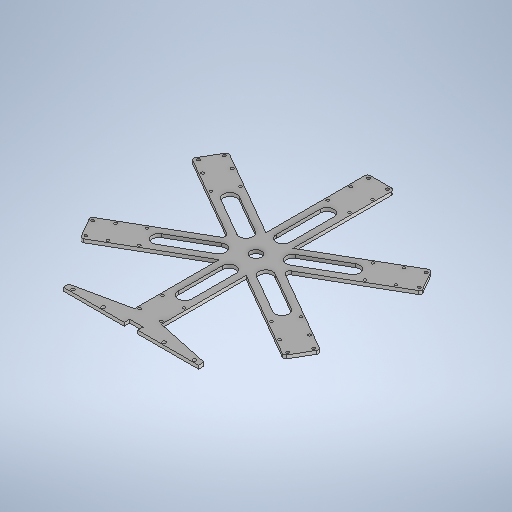
# Autodesk Inventor part: 03
Saved by Autodesk Inventor 2025.1 (Build 291241000, 241)
## iProperties
Created: 2024-09-17
Part Number: 03
Material: Generisch
Document SubType Name: Modeling
Designer: ffogue
Density: 1 g/cm^3
Appearance: Vorgabe
Author: ffogue
Autodesk Inventor part; units mm, degrees
ref_plane "YZ Plane" through (0, 0, 0) normal (1, 0, 0) x (0, 1, 0)
ref_plane "XZ Plane" through (0, 0, 0) normal (0, 1, 0) x (-1, 0, 0)
ref_plane "XY Plane" through (0, 0, 0) normal (0, 0, 1) x (1, 0, 0)
sketch "Sketch1" plane through (0, 0, 0) normal (0, 0, 1) x (1, 0, 0)
  line L0 (-100, 0) -> (-100, -8)
  line L1 (-100, -8) -> (100, -8)
  line L2 (100, -8) -> (100, 0)
  line L3 (0, 0) -> (0, 177) construction
  line L4 (0, 177) -> (82.7625, 129.217) construction
  line L5 (0, 177) -> (-160.2147, 269.5) construction
  line L6 (0, 177) -> (160.2147, 269.5) construction
  line L7 (0, 177) -> (0, 205.8158) construction
  line L8 (0, 177) -> (-85.2909, 127.7573) construction
  line L9 (94.0747, 177) -> (-94.0747, 177) construction
  circle A0 centre (0, 177) radius 40 construction
  line L10 (0, 137) -> (0, 72) construction
  line L11 (10, 137) -> (10, 72)
  line L12 (-10, 72) -> (-10, 137)
  arc A1 (10, 137) -> (-10, 137) centre (0, 137) ccw
  arc A2 (-10, 72) -> (10, 72) centre (0, 72) ccw
  line L13 (-34.641, 157) -> (-90.9327, 124.5) construction
  line L14 (-39.641, 165.6603) -> (-95.9327, 133.1603)
  line L15 (-85.9327, 115.8397) -> (-29.641, 148.3397)
  arc A3 (-29.641, 148.3397) -> (-39.641, 165.6603) centre (-34.641, 157) ccw
  arc A4 (-95.9327, 133.1603) -> (-85.9327, 115.8397) centre (-90.9327, 124.5) ccw
  line L16 (-34.641, 197) -> (-90.9327, 229.5) construction
  line L17 (-39.641, 188.3397) -> (-95.9327, 220.8397)
  line L18 (-85.9327, 238.1603) -> (-29.641, 205.6603)
  arc A5 (-39.641, 188.3397) -> (-29.641, 205.6603) centre (-34.641, 197) ccw
  arc A6 (-85.9327, 238.1603) -> (-95.9327, 220.8397) centre (-90.9327, 229.5) ccw
  line L19 (0, 217) -> (0, 282) construction
  line L20 (10, 217) -> (10, 282)
  line L21 (-10, 282) -> (-10, 217)
  arc A7 (-10, 217) -> (10, 217) centre (0, 217) ccw
  arc A8 (10, 282) -> (-10, 282) centre (0, 282) ccw
  line L22 (34.641, 197) -> (90.9327, 229.5) construction
  line L23 (39.641, 188.3397) -> (95.9327, 220.8397)
  line L24 (85.9327, 238.1603) -> (29.641, 205.6603)
  arc A9 (29.641, 205.6603) -> (39.641, 188.3397) centre (34.641, 197) ccw
  arc A10 (95.9327, 220.8397) -> (85.9327, 238.1603) centre (90.9327, 229.5) ccw
  line L25 (34.641, 157) -> (90.9327, 124.5) construction
  line L26 (29.641, 148.3397) -> (85.9327, 115.8397)
  line L27 (95.9327, 133.1603) -> (39.641, 165.6603)
  arc A11 (39.641, 165.6603) -> (29.641, 148.3397) centre (34.641, 157) ccw
  arc A12 (85.9327, 115.8397) -> (95.9327, 133.1603) centre (90.9327, 124.5) ccw
  circle A13 centre (0, 177) radius 105 construction
  line L28 (-20, 17) -> (-20, 142.359)
  line L29 (-20, 17) -> (-100, 0)
  line L30 (20, 17) -> (20, 142.359)
  line L31 (20, 17) -> (100, 0)
  arc A14 (-20, 142.359) -> (-20, 142.359) centre (-17.5, 138.0289) ccw
  line L32 (-20, 142.359) -> (-150.2147, 67.1795)
  line L33 (-150.2147, 67.1795) -> (-170.2147, 101.8205)
  line L34 (-170.2147, 101.8205) -> (-47.5, 172.6699)
  arc A15 (-47.5, 172.6699) -> (-47.5, 181.3301) centre (-50, 177) ccw
  line L35 (-170.2147, 252.1795) -> (-150.2147, 286.8205)
  arc A16 (-20, 211.641) -> (-20, 211.641) centre (-25, 211.641) ccw
  line L36 (-20, 211.641) -> (-20, 362)
  line L37 (-20, 362) -> (20, 362)
  line L38 (20, 362) -> (20, 211.641)
  line L39 (20, 211.641) -> (150.2147, 286.8205)
  line L40 (150.2147, 286.8205) -> (170.2147, 252.1795)
  line L41 (170.2147, 252.1795) -> (47.5, 181.3301)
  arc A17 (47.5, 181.3301) -> (47.5, 172.6699) centre (50, 177) ccw
  line L42 (47.5, 172.6699) -> (170.2147, 101.8205)
  line L43 (-170.2147, 252.1795) -> (-47.5, 181.3301)
  line L44 (-20, 211.641) -> (-150.2147, 286.8205)
  arc A18 (20, 142.359) -> (20, 142.359) centre (25, 142.359) ccw
  line L45 (20, 142.359) -> (150.2147, 67.1795)
  line L46 (150.2147, 67.1795) -> (170.2147, 101.8205)
  line L47 (0, 177) -> (160.2147, 84.5) construction
  line L48 (-10, -8) -> (-10, 0)
  line L49 (-10, 0) -> (10, 0)
  line L50 (10, 0) -> (10, -8)
  point P0 (0, 104.5)
  point P1 (-62.7868, 140.75)
  point P2 (-62.7868, 213.25)
  point P3 (0, 249.5)
  point P4 (62.7868, 213.25)
  point P5 (62.7868, 140.75)
  point P6 (20, 211.641)
  point P7 (-160.2147, 84.5)
  point P8 (0, 0)
  dimension "d10" = 80
  dimension "d0" = 200
  dimension "d1" = 8
  dimension "d4" = 60
  dimension "d6" = 60
  dimension "d7" = 60
  dimension "d8" = 60
  dimension "d9" = 185
  dimension "d11" = 10
  dimension "d12" = 10
  dimension "d13" = 10
  dimension "d14" = 10
  dimension "d15" = 10
  dimension "d16" = 10
  dimension "d17" = 210
  dimension "d19" = 25
  dimension "d20" = 25
  dimension "d21" = 5
  dimension "d22" = 90
  dimension "d25" = 5
  dimension "d30" = 185
  dimension "d32" = 185
  dimension "d33" = 185
  dimension "d34" = 5
  dimension "d35" = 185
  dimension "d36" = 5
  dimension "d39" = 5
  dimension "d40" = 185
  dimension "d43" = 8
  dimension "d44" = 20
  dimension "d84" = 40
  dimension "d85" = 40
  dimension "d86" = 40
  dimension "d87" = 40
  dimension "d114" = 40
  constraints: 114 end point, 40 point on circle, 30 tangent, 18 centre point, 16 parallel, 14 point on line, 12 midpoint, 8 vertical, 6 perpendicular, 5 horizontal alignment, 3 coincident, 2 horizontal, 21 other
  measures "d0" distance of L0.end L1.end
  measures "d1" distance of L0.start L0.end
  measures "d4" angle of L4 L3
  measures "d6" angle of L6 L7
  measures "d7" angle of L3 L8
  measures "d8" angle of L7 L5
  measures "d9" distance from line of L3.end L1
  measures "d11" radius of A3
  measures "d12" radius of A1
  measures "d13" radius of A11
  measures "d14" radius of A9
  measures "d15" radius of A7
  measures "d16" radius of A5
  measures "d17" diameter of A13
  measures "d19" vertical distance of L30.start L1.end
  measures "d20" distance from line of L28.start L1
  measures "d21" radius of A14
  measures "d22" angle of L32 L33
  measures "d25" radius of A15
  measures "d30" distance from line of L9 L36.end
  measures "d32" distance of L5.end L3.end
  measures "d33" distance of point (-160.215, 84.5) A13.centre
  measures "d34" radius of A16
  measures "d35" distance of L3.end L6.end
  measures "d36" radius of A17
  measures "d39" radius of A18
  measures "d40" distance of L47.end L3.end
  measures "d43" distance between parallel lines of L1 L49
  measures "d44" distance of L48.end L49.end
  measures "d84" distance between parallel lines of L32 L34
  measures "d85" distance between parallel lines of L44 L43
  measures "d86" distance between parallel lines of L38 L36
  measures "d87" distance between parallel lines of L41 L39
  measures "d114" distance between parallel lines of L30 L28
extrude "Extrusion2" add sketch "Sketch1" along normal mid plane 5 contours L29 L28 A14 L32 L33 L34 A15 L43 L35 L44 A16 L36 L37 L38 L39 L40 L41 A17 L42 L46 L45 A18 L30 L31 L2 L1 L50 L49 L48 L0 | L28 A14 | A18 L45 | L44 A16 picked at (-17.1896, 138.26) picked at (23.5757, 142.474) picked at (-23.6127, 211.5125)
sketch "Sketch3" plane through (0, 0, 2.5) normal (0, 0, 1) x (1, 0, 0)
  line L0 (-100, -8) -> (-10, -8) projected
  line L1 (-10, -8) -> (-10, 0) projected
  line L2 (-10, 0) -> (10, 0) projected
  line L3 (10, 0) -> (10, -8) projected
  line L4 (10, -8) -> (100, -8) projected
  line L5 (100, -8) -> (100, 0) projected
  line L6 (100, 0) -> (20, 17) projected
  line L7 (20, 17) -> (20, 142.359) projected
  line L8 (20, 142.359) -> (150.2147, 67.1795) projected
  line L9 (150.2147, 67.1795) -> (170.2147, 101.8205) projected
  line L10 (170.2147, 101.8205) -> (47.5, 172.6699) projected
  arc A0 (47.5, 181.3301) -> (47.5, 172.6699) centre (50, 177) ccw projected
  line L11 (47.5, 181.3301) -> (170.2147, 252.1795) projected
  line L12 (170.2147, 252.1795) -> (150.2147, 286.8205) projected
  line L13 (150.2147, 286.8205) -> (20, 211.641) projected
  line L14 (20, 211.641) -> (20, 362) projected
  line L15 (20, 362) -> (-20, 362) projected
  line L16 (-20, 362) -> (-20, 211.641) projected
  line L17 (-20, 211.641) -> (-150.2147, 286.8205) projected
  line L18 (-150.2147, 286.8205) -> (-170.2147, 252.1795) projected
  line L19 (-170.2147, 252.1795) -> (-47.5, 181.3301) projected
  arc A1 (-47.5, 172.6699) -> (-47.5, 181.3301) centre (-50, 177) ccw projected
  line L20 (-47.5, 172.6699) -> (-170.2147, 101.8205) projected
  line L21 (-170.2147, 101.8205) -> (-150.2147, 67.1795) projected
  line L22 (-150.2147, 67.1795) -> (-20, 142.359) projected
  line L23 (-20, 142.359) -> (-20, 17) projected
  line L24 (-20, 17) -> (-100, 0) projected
  line L25 (-100, 0) -> (-100, -8) projected
  arc A2 (39.641, 165.6603) -> (29.641, 148.3397) centre (34.641, 157) ccw projected
  line L26 (39.641, 165.6603) -> (95.9327, 133.1603) projected
  arc A3 (85.9327, 115.8397) -> (95.9327, 133.1603) centre (90.9327, 124.5) ccw projected
  line L27 (85.9327, 115.8397) -> (29.641, 148.3397) projected
  arc A4 (29.641, 205.6603) -> (39.641, 188.3397) centre (34.641, 197) ccw projected
  line L28 (29.641, 205.6603) -> (85.9327, 238.1603) projected
  arc A5 (95.9327, 220.8397) -> (85.9327, 238.1603) centre (90.9327, 229.5) ccw projected
  line L29 (95.9327, 220.8397) -> (39.641, 188.3397) projected
  arc A6 (-10, 217) -> (10, 217) centre (0, 217) ccw projected
  line L30 (-10, 217) -> (-10, 282) projected
  arc A7 (10, 282) -> (-10, 282) centre (0, 282) ccw projected
  line L31 (10, 282) -> (10, 217) projected
  line L32 (-85.9327, 238.1603) -> (-29.641, 205.6603) projected
  arc A8 (-39.641, 188.3397) -> (-29.641, 205.6603) centre (-34.641, 197) ccw projected
  line L33 (-39.641, 188.3397) -> (-95.9327, 220.8397) projected
  arc A9 (-85.9327, 238.1603) -> (-95.9327, 220.8397) centre (-90.9327, 229.5) ccw projected
  arc A10 (-29.641, 148.3397) -> (-39.641, 165.6603) centre (-34.641, 157) ccw projected
  line L34 (-29.641, 148.3397) -> (-85.9327, 115.8397) projected
  arc A11 (-95.9327, 133.1603) -> (-85.9327, 115.8397) centre (-90.9327, 124.5) ccw projected
  line L35 (-95.9327, 133.1603) -> (-39.641, 165.6603) projected
  line L36 (-10, 72) -> (-10, 137) projected
  arc A12 (10, 137) -> (-10, 137) centre (0, 137) ccw projected
  line L37 (10, 137) -> (10, 72) projected
  arc A13 (-10, 72) -> (10, 72) centre (0, 72) ccw projected
  line L38 (-50, 177) -> (50, 177) construction
  line L39 (0, 217) -> (0, 137) construction
  circle A14 centre (0, 177) radius 123 construction
  circle A15 centre (0, 177) radius 157 construction
  circle A16 centre (0, 177) radius 181 construction
  point P0 (0, 0)
  point P1 (14, 20)
  point P2 (14, 54)
  point P3 (-14, 20)
  point P4 (-14, 54)
  point P5 (55, -8)
  point P6 (-14, 299.2007)
  point P7 (14, 299.2007)
  point P8 (-14, 333.3746)
  point P9 (14, 333.3746)
  point P10 (-14, 357.4578)
  point P11 (14, 357.4578)
  dimension "d47" = 246
  dimension "d48" = 314
  dimension "d49" = 362
  dimension "d50" = 28
  dimension "d51" = 34
  dimension "d52" = 14
  dimension "d53" = 28
  dimension "d54" = 14
  dimension "d55" = 28
  constraints: 6 coincident, 6 point on circle, 5 midpoint, 5 vertical alignment, 4 end point, 4 horizontal alignment, 3 centre point, 1 vertical
  measures "d47" diameter of A14
  measures "d48" diameter of A15
  measures "d49" diameter of A16
  measures "d50" vertical distance of point (55, -8) point (14, 20)
  measures "d51" distance of point (14, 54) point (14, 20)
  measures "d52" horizontal distance of A13.centre point (-14, 54)
  measures "d53" distance of point (14, 54) point (-14, 54)
  measures "d54" horizontal distance of A7.centre A16.start
  measures "d55" distance of A16.end A16.start
fillet "Fillet1" radius 4 10 edges at (20, 362, 0) (-20, 362, 0) (150.2147, 286.8205, 0) (170.2147, 252.1795, 0) (170.2147, 101.8205, 0) (150.2147, 67.1795, 0) (-150.2147, 67.1795, 0) (-170.2147, 101.8205, 0) (-170.2147, 252.1795, 0) (-150.2147, 286.8205, 0)
sketch "Sketch4" plane through (0, 0, 2.5) normal (0, 0, 1) x (1, 0, 0)
  circle A0 centre (0, 177) radius 8
  arc A1 (-47.5, 172.6699) -> (-47.5, 181.3301) centre (-50, 177) ccw projected
  arc A2 (47.5, 181.3301) -> (47.5, 172.6699) centre (50, 177) ccw projected
  point P0 (0, 0)
  dimension "d79" = 16
  constraints: 1 centre point, 1 horizontal alignment, 1 vertical alignment
  measures "d79" diameter of A0
extrude "Extrusion3" cut sketch "Sketch4" against normal up to surface (5 mm away)
sketch "Sketch5" plane through (0, 0, 2.5) normal (0, 0, 1) x (1, 0, 0)
  line L0 (16, 362) -> (-16, 362) projected
  circle A0 centre (0, 177) radius 8 projected
  circle A1 centre (0, 177) radius 181 construction
  line L1 (-152.2147, 283.3564) -> (-168.2147, 255.6436) projected
  line L2 (0, 177) -> (-163.8744, 82.3871) construction
  line L3 (-168.2147, 98.3564) -> (-152.2147, 70.6436) projected
  line L4 (-146.7506, 69.1795) -> (-20, 142.359) projected
  line L5 (0, 177) -> (162.5999, 83.1229) construction
  line L6 (-39.641, 188.3397) -> (-95.9327, 220.8397) projected
  line L7 (166.7506, 103.8205) -> (47.5, 172.6699) projected
  point P0 (0, 0)
  point P1 (-14, 357.4578)
  point P2 (14, 357.4578)
  point P3 (0, 362)
  point P4 (-163.281, 255.1045)
  point P5 (-149.281, 279.3532)
  point P6 (-163.281, 98.8955)
  point P7 (-149.281, 74.6468)
  point P8 (149.281, 74.6468)
  point P9 (163.281, 98.8955)
  point P10 (149.281, 279.3532)
  point P11 (163.281, 255.1045)
  point P12 (-160.2147, 269.5)
  dimension "d88" = 362
  dimension "d82" = 28
  dimension "d83" = 14
  dimension "d91" = 28
  dimension "d92" = 28
  dimension "d93" = 28
  dimension "d101" = 28
  constraints: 4 end point, 4 symmetric about line, 3 parallel, 2 midpoint, 1 coincident, 1 horizontal alignment, 1 perpendicular, 11 other
  measures "d82" distance of point (14, 357.458) point (-14, 357.458)
  measures "d83" horizontal distance of point (0, 362) point (-14, 357.458)
  measures "d91" distance of point (-149.281, 74.647) point (-163.281, 98.895)
  measures "d92" distance of point (163.281, 255.105) point (149.281, 279.353)
  measures "d93" distance of point (163.281, 98.895) point (149.281, 74.647)
  measures "d101" distance of point (-149.281, 279.353) point (-163.281, 255.105)
hole "Hole4" at (-14, 357.4578, 2.5) at (14, 357.4578, 2.5) at (-163.281, 255.1045, 2.5) at (-149.281, 279.3532, 2.5) at (-163.281, 98.8955, 2.5) at (-149.281, 74.6468, 2.5) at (149.281, 74.6468, 2.5) at (163.281, 98.8955, 2.5) at (149.281, 279.3532, 2.5) at (163.281, 255.1045, 2.5) direction (0, 0, -1) diameter 4.134 depth 5 thread size "M5x0.8" class "6H" standard "ISO Metric profile"
sketch "Sketch6" plane through (0, 0, 2.5) normal (0, 0, 1) x (1, 0, 0)
  circle A0 centre (0, 177) radius 8 projected
  circle A1 centre (0, 177) radius 8 projected
  circle A2 centre (0, 177) radius 157 construction
  line L0 (-168.2147, 98.3564) -> (-152.2147, 70.6436) projected
  line L1 (-160.2147, 84.5) -> (156.816, 267.5378) construction
  line L2 (-146.7506, 69.1795) -> (-20, 142.359) projected
  line L3 (152.2147, 70.6436) -> (168.2147, 98.3564) projected
  line L4 (160.2147, 84.5) -> (-161.7662, 270.3958) construction
  line L5 (-20, 211.641) -> (-146.7506, 284.8205) projected
  line L6 (16, 362) -> (-16, 362) projected
  line L7 (-10, 0) -> (10, 0) projected
  line L8 (0, 0) -> (0, 362) construction
  line L9 (10, 217) -> (10, 282) projected
  point P0 (0, 0)
  point P1 (-143.2581, 241.2349)
  point P2 (-127.2581, 268.9477)
  point P3 (-16, 333.1826)
  point P4 (16, 333.1826)
  point P5 (127.2581, 268.9477)
  point P6 (143.2581, 241.2349)
  point P7 (143.2581, 112.7651)
  point P8 (127.2581, 85.0523)
  point P9 (16, 20.8174)
  point P10 (-16, 20.8174)
  point P11 (-16, 54.8174)
  point P12 (16, 54.8174)
  point P13 (-127.2581, 85.0523)
  point P14 (-143.2581, 112.7651)
  point P15 (-21.4634, 210.7539)
  point P16 (-146.7506, 284.8205)
  point P17 (-97.8132, 102.0523)
  point P18 (-113.8132, 129.7651)
  point P19 (-113.8132, 224.2349)
  point P20 (-97.8132, 251.9477)
  point P21 (-16, 299.1826)
  point P22 (16, 299.1826)
  point P23 (97.8132, 251.9477)
  point P24 (113.8132, 224.2349)
  point P25 (113.8132, 129.7651)
  point P26 (97.8132, 102.0523)
  dimension "d102" = 314
  dimension "d104" = 32
  dimension "d105" = 16
  dimension "d106" = 32
  dimension "d107" = 32
  dimension "d108" = 16
  dimension "d109" = 32
  dimension "d110" = 16
  dimension "d111" = 32
  dimension "d112" = 32
  dimension "d113" = 16
  dimension "d117" = 32
  dimension "d118" = 32
  dimension "d119" = 32
  dimension "d120" = 32
  dimension "d121" = 32
  dimension "d141" = 34
  dimension "d142" = 34
  dimension "d143" = 34
  dimension "d144" = 34
  dimension "d145" = 34
  dimension "d146" = 34
  constraints: 7 symmetric about line, 6 end point, 4 midpoint, 3 vertical alignment, 2 parallel, 1 coincident, 1 horizontal alignment, 16 other
  measures "d104" distance of point (-16, 20.817) point (16, 20.817)
  measures "d105" horizontal distance of point (0, 0) point (-16, 20.817)
  measures "d106" distance of point (-143.258, 112.765) point (-127.258, 85.052)
  measures "d107" distance of point (-127.258, 268.948) point (-143.258, 241.235)
  measures "d108" distance from line of L4 point (-143.258, 241.235)
  measures "d109" distance of point (16, 333.183) point (-16, 333.183)
  measures "d110" horizontal distance of L8.end point (-16, 333.183)
  measures "d111" distance of point (143.258, 241.235) point (127.258, 268.948)
  measures "d112" distance of point (127.258, 85.052) point (143.258, 112.765)
  measures "d113" distance from line of L4 point (143.258, 112.765)
  measures "d117" distance of point (-97.813, 251.948) point (-113.813, 224.235)
  measures "d118" distance of point (16, 299.183) point (-16, 299.183)
  measures "d119" distance of point (113.813, 224.235) point (97.813, 251.948)
  measures "d120" distance of point (113.813, 129.765) point (97.813, 102.052)
  measures "d121" distance of point (-113.813, 129.765) point (-97.813, 102.052)
  measures "d141" distance of point (-16, 333.183) point (-16, 299.183)
  measures "d142" distance of point (-127.258, 268.948) point (-97.813, 251.948)
  measures "d143" distance of point (-143.258, 112.765) point (-113.813, 129.765)
  measures "d144" distance of point (-16, 20.817) point (-16, 54.817)
  measures "d145" distance of point (143.258, 241.235) point (113.813, 224.235)
  measures "d146" distance of point (143.258, 112.765) point (113.813, 129.765)
hole "Hole5" at (-143.2581, 241.2349, 2.5) at (-127.2581, 268.9477, 2.5) at (-16, 333.1826, 2.5) at (16, 333.1826, 2.5) at (127.2581, 268.9477, 2.5) at (143.2581, 241.2349, 2.5) at (143.2581, 112.7651, 2.5) at (127.2581, 85.0523, 2.5) at (16, 20.8174, 2.5) at (-16, 20.8174, 2.5) at (-16, 54.8174, 2.5) at (16, 54.8174, 2.5) at (-127.2581, 85.0523, 2.5) at (-143.2581, 112.7651, 2.5) at (-97.8132, 102.0523, 2.5) at (-113.8132, 129.7651, 2.5) at (-113.8132, 224.2349, 2.5) at (-97.8132, 251.9477, 2.5) at (-16, 299.1826, 2.5) at (16, 299.1826, 2.5) at (97.8132, 251.9477, 2.5) at (113.8132, 224.2349, 2.5) at (113.8132, 129.7651, 2.5) at (97.8132, 102.0523, 2.5) direction (0, 0, -1) diameter 4 depth 5
sketch "Sketch7" plane through (0, 0, 2.5) normal (0, 0, 1) x (1, 0, 0)
  line L0 (-10, 0) -> (10, 0) projected
  line L1 (-100, -8) -> (-10, -8) projected
  point P0 (0, 0)
  point P1 (-90, -4)
  point P2 (-45, -4)
  point P3 (45, -4)
  point P4 (90, -4)
  point P5 (0, 0)
  dimension "d129" = 180
  dimension "d130" = 45
  dimension "d131" = 45
  dimension "d132" = 45
  dimension "d133" = 4
  constraints: 3 horizontal alignment, 1 midpoint
  measures "d129" distance of point (90, -4) point (-90, -4)
  measures "d130" distance of point (-45, -4) point (-90, -4)
  measures "d131" distance of point (90, -4) point (45, -4)
  measures "d132" horizontal distance of point (0, 0) point (-45, -4)
  measures "d133" distance from line of L1 point (-90, -4)
hole "Hole6" at (-90, -4, 2.5) at (-45, -4, 2.5) at (45, -4, 2.5) at (90, -4, 2.5) direction (0, 0, -1) diameter 5 depth 5
sketch "Sketch8" plane through (0, 0, 2.5) normal (0, 0, 1) x (1, 0, 0)
  circle A0 centre (0, 177) radius 8 projected
  circle A1 centre (0, 177) radius 13
  circle A2 centre (0, 177) radius 8 projected
  point P0 (0, 0)
  dimension "d147" = 26
  constraints: 1 centre point, 1 coincident
  measures "d147" diameter of A1
equation "\"d6\" = d4"
equation "\"d7\" = d4"
equation "\"d8\" = d4"
equation "\"d12\" = d11"
equation "\"d13\" = d11"
equation "\"d14\" = d11"
equation "\"d15\" = d11"
equation "\"d16\" = d11"
equation "\"d32\" = d30"
equation "\"d34\" = d25"
equation "\"d52\" = 0.5 * d53"
equation "\"d83\" = 0.5 * d82"
body "Solid2"
